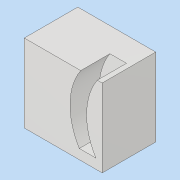
# Autodesk Inventor part: limitSwitchTab
Saved by Autodesk Inventor 2017 (Build 210142000, 142)
## iProperties
Created: 2019-07-12
Part Number: limitSwitchTab
Material: ABS Plastic
Document SubType Name: Modeling
Designer: techn
Density: 1.06 g/cm^3
Appearance: Smooth - White
Author: techn
Autodesk Inventor part; units mm, degrees
ref_plane "YZ Plane" through (0, 0, 0) normal (1, 0, 0) x (0, 1, 0)
ref_plane "XZ Plane" through (0, 0, 0) normal (0, 1, 0) x (-1, 0, 0)
ref_plane "XY Plane" through (0, 0, 0) normal (0, 0, 1) x (1, 0, 0)
sketch "Sketch1" plane through (0, 0, 0) normal (0, 0, 1) x (1, 0, 0)
  line L0 (0, 0) -> (10.16, 0)
  line L1 (10.16, 0) -> (10.16, 10.16)
  line L2 (10.16, 10.16) -> (0, 10.16)
  line L3 (0, 10.16) -> (0, 0)
  dimension "d0" = 10.16
  dimension "d1" = 10.16
  constraints: 8 end point, 2 parallel, 1 horizontal, 1 perpendicular
  measures "d0" distance of L1.end L2.end
  measures "d1" distance of L0.end L1.end
extrude "Extrusion1" add sketch "Sketch1" along normal blind 6.985
sketch "Sketch2" plane through (0, 0, 6.985) normal (0, 0, 1) x (1, 0, 0)
  line L0 (0, 0) -> (10.16, 0) construction
  line L1 (10.16, 0) -> (10.16, 10.16) construction
  line L2 (10.16, 10.16) -> (0, 10.16) construction
  line L3 (0, 10.16) -> (0, 0) construction
  arc A0 (9.525, 10.16) -> (9.3363, 1.27) centre (16.3845, 5.5674) ccw
  arc A1 (7.3607, 10.16) -> (7.172, 1.27) centre (14.2202, 5.5674) ccw
  line L4 (7.3607, 10.16) -> (9.525, 10.16)
  line L5 (10.16, 10.16) -> (0, 10.16) projected
  line L6 (7.172, 1.27) -> (9.3363, 1.27)
  dimension "d4" = 8.255
  dimension "d5" = 0.635
  dimension "d6" = 1.27
  constraints: 4 end point, 4 point on circle, 2 centre point, 2 point on line, 1 collinear, 1 equal radius, 1 horizontal, 1 horizontal alignment
  measures "d4" radius of A0
  measures "d5" distance of L4.end L1.end
  measures "d6" distance between parallel lines of L0 L6
extrude "Extrusion2" cut sketch "Sketch2" against normal blind 3.81
body "Solid1"
